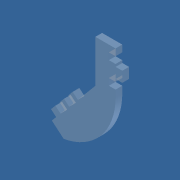
# Autodesk Inventor part: acrylic kinect bracket - bracket
Saved by Autodesk Inventor 2012 (Build 160160000, 160)
## iProperties
Created: 2012-10-30
Part Number: acrylic kinect bracket - bracket
Material: Default
Document SubType Name: Modeling
Designer: Ed
Density: 1 g/cm^3
Author: Ed
Autodesk Inventor part; units mm, degrees
ref_plane "YZ Plane" through (0, 0, 0) normal (1, 0, 0) x (0, 1, 0)
ref_plane "XZ Plane" through (0, 0, 0) normal (0, 1, 0) x (-1, 0, 0)
ref_plane "XY Plane" through (0, 0, 0) normal (0, 0, 1) x (1, 0, 0)
sketch "Sketch1" plane through (0, 0, 0) normal (0, 0, 1) x (1, 0, 0)
  line L0 (-19.05, -20) -> (-60.1594, -68.9923)
  line L1 (-6.35, -7.3) -> (0, -7.3)
  line L2 (0, -7.3) -> (0, -13.65)
  line L3 (0, -13.65) -> (-6.35, -13.65)
  line L4 (-6.35, -13.65) -> (-6.35, -7.3)
  line L5 (6.35, -4.953) -> (0, -4.953)
  line L6 (0, -4.953) -> (0, 4.953)
  line L7 (0, 4.953) -> (6.35, 4.953)
  line L8 (6.35, 4.953) -> (6.35, -4.953)
  line L9 (-6.35, 13.65) -> (0, 13.65)
  line L10 (0, 13.65) -> (0, 7.3)
  line L11 (0, 7.3) -> (-6.35, 7.3)
  line L12 (-6.35, 7.3) -> (-6.35, 13.65)
  line L13 (0, -20) -> (-19.05, -20)
  line L14 (-19.05, -20) -> (-19.05, 20)
  line L15 (-19.05, 20) -> (0, 20)
  line L16 (0, 20) -> (0, -20)
  line L17 (-48.9804, -78.3726) -> (-8.1634, -29.7288)
  line L18 (-8.1634, -29.7288) -> (0, -20)
  line L19 (-48.9804, -78.3726) -> (-60.1594, -68.9923)
  line L20 (-56.0777, -64.1279) -> (-51.996, -59.2635)
  line L21 (-51.996, -59.2635) -> (-56.8604, -55.1818)
  line L22 (-56.8604, -55.1818) -> (-60.9421, -60.0462)
  line L23 (-60.9421, -60.0462) -> (-56.0777, -64.1279)
  line L24 (-47.9143, -54.3991) -> (-43.8326, -49.5348)
  line L25 (-43.8326, -49.5348) -> (-48.697, -45.4531)
  line L26 (-48.697, -45.4531) -> (-52.7787, -50.3174)
  line L27 (-52.7787, -50.3174) -> (-47.9143, -54.3991)
  line L28 (-39.7509, -44.6704) -> (-35.6692, -39.806)
  line L29 (-35.6692, -39.806) -> (-40.5336, -35.7243)
  line L30 (-40.5336, -35.7243) -> (-44.6153, -40.5887)
  line L31 (-44.6153, -40.5887) -> (-39.7509, -44.6704)
  arc A0 (-48.9804, -78.3726) -> (0, -20) centre (-59.2731, -20) ccw
  point P0 (0, 0)
  point P1 (0, 0)
  dimension "d0" = 6.35
  dimension "d2" = 9.906
  dimension "d3" = 40
  dimension "d4" = 6.35
  dimension "d5" = 6.35
  dimension "d6" = 6.35
  dimension "d10" = 50
  dimension "d11" = 19.05
  dimension "d12" = 12.7
  dimension "d15" = 6.35
  dimension "d16" = 6.35
  dimension "d19" = 12.7
  dimension "d24" = 76.2
  constraints: 64 end point, 10 parallel, 6 perpendicular, 4 collinear, 4 equal length, 4 horizontal, 2 midpoint, 2 point on circle, 2 point on line, 1 centre point, 1 coincident, 1 tangent, 17 other
  measures "d0" distance of L9.end L10.end
  measures "d2" distance of L7.end L5.start
  measures "d3" distance of L15.end L13.start
  measures "d4" distance of L6.end L7.end
  measures "d5" distance between parallel lines of L15 L9
  measures "d6" distance between parallel lines of L13 L3
  measures "d10" angle of L13 L18
  measures "d11" distance of L14.end L15.end
  measures "d12" distance of L17.end L13.start
  measures "d15" distance of L22.end L20.start
  measures "d16" distance between parallel lines of L19 L23
  measures "d19" distance of L20.end L25.start
  measures "d24" distance from line of L13.start L19
extrude "Extrusion1" add sketch "Sketch1" along normal blind 6.35 contours L13 L18 L17 L19 L0 | L14 L15 L16 L9 L12 L11 L6 L1 L4 L3 L13 | L0 L31 L30 L29 | A0 L17 L18 | L0 L27 L26 L25 | L6 L7 L8 L5 | L23 L22 L21 L0
body "Solid1"
